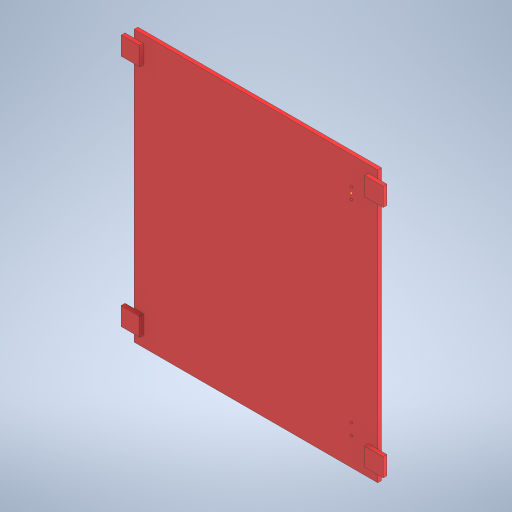
# Autodesk Inventor part: superficie
Saved by Autodesk Inventor 2023.2 (Build 272271030, 271C)
## iProperties
Created: 2023-03-05
Part Number: superficie
Material: Generic
Document SubType Name: Sheet Metal
Designer: angel
Density: 1 g/cm^3
Sheet Metal Rule: Default_mm
Appearance: Default
Author: angel
Autodesk Inventor part; units mm, degrees
ref_plane "YZ Plane" through (0, 0, 0) normal (1, 0, 0) x (0, 1, 0)
ref_plane "XZ Plane" through (0, 0, 0) normal (0, 1, 0) x (-1, 0, 0)
ref_plane "XY Plane" through (0, 0, 0) normal (0, 0, 1) x (1, 0, 0)
sketch "Sketch1" plane through (0, 0, 0) normal (0, 0, 1) x (1, 0, 0)
  line L0 (-589.5801, 90.5) -> (-589.5801, -645.2993)
  line L1 (-589.5801, -645.2993) -> (-564.1801, -645.2993)
  line L2 (-589.5801, 90.5) -> (-564.1801, 90.5)
  line L3 (71.6192, 90.5) -> (46.2192, 90.5)
  line L4 (71.6192, -645.2993) -> (71.6192, 90.5)
  line L5 (71.6192, -645.2993) -> (46.2192, -645.2993)
  circle A0 centre (0, -569.7993) radius 2.55
  circle A1 centre (0, -539.7993) radius 2.55
  circle A2 centre (0, -15) radius 2.55
  circle A3 centre (0, 15) radius 2.55
  line L6 (-589.5801, -645.2993) -> (-589.5801, 90.5)
  line L7 (-589.5801, 90.5) -> (71.6192, 90.5)
  line L8 (71.6192, 90.5) -> (71.6192, -645.2993)
  line L9 (71.6192, -645.2993) -> (-589.5801, -645.2993)
  circle A4 centre (0, -569.7993) radius 2.55
  circle A5 centre (0, -539.7993) radius 2.55
  circle A6 centre (0, -15) radius 2.55
  circle A7 centre (0, 15) radius 2.55
  circle A8 centre (58.9192, -595.2991) radius 2.55
  circle A9 centre (58.9192, 40.4999) radius 2.55
  circle A10 centre (-576.8801, 40.4999) radius 2.55
  circle A11 centre (-576.8801, -595.2991) radius 2.55
  point P0 (0, 0)
  point P1 (58.9192, -645.2993)
  point P2 (-576.8801, 90.5)
  point P3 (71.6192, -277.3996)
  point P4 (71.6192, -277.3996)
  dimension "d0" = 735.7993
  dimension "d3" = 5.1
  dimension "d12" = 635.799
  dimension "d13" = 317.8995
  measures "d0" distance of L4.start L3.start
  measures "d3" diameter of A9
  measures "d12" distance of A9.centre A8.centre
  measures "d13" vertical distance of A9.centre point (71.619, -277.4)
extrude "Plate1" add sketch "Sketch1" along normal blind 10
sketch "Sketch2" plane through (0, 0, 10) normal (0, 0, 1) x (1, 0, 0)
  point P0 (0, 0)
sketch "Sketch3" plane through (0, 0, 10) normal (0, 0, 1) x (1, 0, 0)
  line L0 (71.6192, 90.5) -> (71.6192, -645.2993) construction
  line L1 (-589.5801, -645.2993) -> (-589.5801, 90.5) construction
  line L2 (46.6192, 19.4621) -> (96.6192, 19.4621)
  line L3 (96.6192, 19.4621) -> (96.6192, 69.4621)
  line L4 (96.6192, 69.4621) -> (46.6192, 69.4621)
  line L5 (46.6192, 69.4621) -> (46.6192, 19.4621)
  line L6 (46.6192, 19.4621) -> (96.6192, 69.4621) construction
  line L7 (96.6192, 19.4621) -> (46.6192, 69.4621) construction
  line L8 (46.6192, -616.3369) -> (96.6192, -616.3369)
  line L9 (96.6192, -616.3369) -> (96.6192, -566.3369)
  line L10 (96.6192, -566.3369) -> (46.6192, -566.3369)
  line L11 (46.6192, -566.3369) -> (46.6192, -616.3369)
  line L12 (46.6192, -616.3369) -> (96.6192, -566.3369) construction
  line L13 (96.6192, -616.3369) -> (46.6192, -566.3369) construction
  line L14 (-614.5801, -616.3369) -> (-564.5801, -616.3369)
  line L15 (-564.5801, -616.3369) -> (-564.5801, -566.3369)
  line L16 (-564.5801, -566.3369) -> (-614.5801, -566.3369)
  line L17 (-614.5801, -566.3369) -> (-614.5801, -616.3369)
  line L18 (-614.5801, -616.3369) -> (-564.5801, -566.3369) construction
  line L19 (-564.5801, -616.3369) -> (-614.5801, -566.3369) construction
  line L20 (-614.5801, 19.4621) -> (-564.5801, 19.4621)
  line L21 (-564.5801, 19.4621) -> (-564.5801, 69.4621)
  line L22 (-564.5801, 69.4621) -> (-614.5801, 69.4621)
  line L23 (-614.5801, 69.4621) -> (-614.5801, 19.4621)
  line L24 (-614.5801, 19.4621) -> (-564.5801, 69.4621) construction
  line L25 (-564.5801, 19.4621) -> (-614.5801, 69.4621) construction
  circle A0 centre (-576.8801, -595.2991) radius 2.55 construction
  circle A1 centre (-576.8801, 40.4999) radius 2.55 construction
  circle A2 centre (58.9192, 40.4999) radius 2.55 construction
  circle A3 centre (58.9192, -595.2991) radius 2.55 construction
  circle A4 centre (0, 15) radius 2.55 construction
  circle A5 centre (0, -15) radius 2.55 construction
  circle A6 centre (0, -539.7993) radius 2.55 construction
  circle A7 centre (0, -569.7993) radius 2.55 construction
  line L26 (-589.5801, 90.5) -> (-589.5801, -645.2993) construction
  line L27 (71.6192, 90.5) -> (-589.5801, 90.5) construction
  line L28 (71.6192, -645.2993) -> (71.6192, 90.5) construction
  line L29 (-589.5801, -645.2993) -> (71.6192, -645.2993) construction
  point P0 (0, 0)
  point P1 (71.6192, 44.4621)
  point P2 (71.6192, -591.3369)
  point P3 (-589.5801, -591.3369)
  point P4 (-589.5801, 44.4621)
  dimension "d5" = 50
  dimension "d11" = 635.799
  constraints: 48 end point, 8 midpoint, 8 parallel, 7 equal length, 5 horizontal alignment, 4 horizontal, 4 perpendicular, 3 vertical alignment, 1 point on line
  measures "d5" distance of L2.end L3.end
  measures "d11" distance of point (-589.58, 44.462) point (-589.58, -591.337)
sheet face with bend "Face2" sketch "Sketch3" thickness 10 toward (0, 0, 1) bend radius 10 relief straight relief width 10 relief depth 5
bend "Bend1"
equation "\"d4\" = Thickness"
equation "\"d6\" = BendRadius"
equation "\"d7\" = BendReliefWidth"
equation "\"d9\" = MinimumRemnant"
equation "\"d8\" = BendReliefDepth"
equation "\"d10\" = TransitionRadius"
equation "\"BendRadius\" = Thickness"
equation "\"BendReliefDepth\" = 0.5 * Thickness"
equation "\"Thickness\" = 10"
equation "\"BendReliefWidth\" = 10"
equation "\"MinimumRemnant\" = 20"
equation "\"TransitionRadius\" = 10"
body "Solid1"
